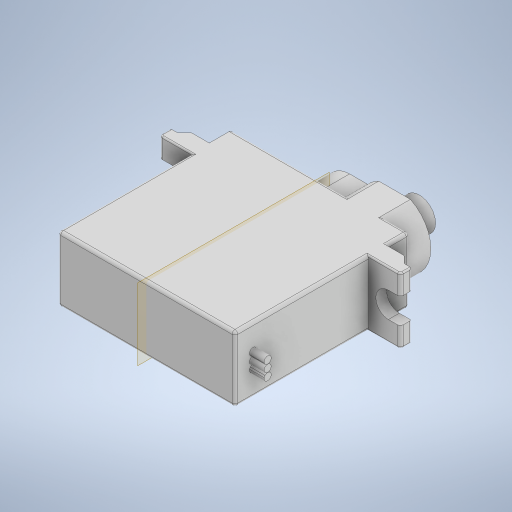
# Autodesk Inventor part: servo_stefan
Saved by Autodesk Inventor 2023 (Build 270158000, 158)
## iProperties
Created: 2023-04-06
Part Number: servo_stefan
Material: Ogólny
Document SubType Name: Modeling
Designer: Kamil
Density: 1 g/cm^3
Appearance: Domyślna
Author: Kamil
Autodesk Inventor part; units mm, degrees
ref_plane "YZ Plane" through (0, 0, 0) normal (1, 0, 0) x (0, 1, 0)
ref_plane "XZ Plane" through (0, 0, 0) normal (0, 1, 0) x (-1, 0, 0)
ref_plane "XY Plane" through (0, 0, 0) normal (0, 0, 1) x (1, 0, 0)
sketch "Szkic1" plane through (0, 0, 0) normal (0, 1, 0) x (-1, 0, 0)
  line L0 (0, 0) -> (24.4, 0)
  line L1 (24.4, 0) -> (24.4, -24)
  line L2 (24.4, -24) -> (0, -24)
  line L3 (0, -24) -> (0, 0)
  dimension "d0" = 24.4
  dimension "d1" = 24
  constraints: 8 end point, 2 parallel, 1 horizontal, 1 perpendicular
  measures "d0" distance of L1.end L2.end
  measures "d1" distance of L0.end L1.end
extrude "Wyciągnięcie proste1" add sketch "Szkic1" along normal blind 9
sketch "Szkic2" plane through (-24.4, 0, -24) normal (-1, 0, 0) x (0, 0, 1)
  line L0 (0, 0) -> (24, 0) projected
  line L1 (24, 0) -> (24, 9) projected
  line L2 (0, 9) -> (24, 9) projected
  line L3 (0, 0) -> (0, 9) projected
  line L4 (24, 0) -> (5.6, 0)
  line L5 (5.6, 0) -> (5.6, 9)
  line L6 (5.6, 9) -> (24, 9)
  line L7 (24, 9) -> (24, 0)
  line L8 (5.6, 9) -> (4.1, 9)
  line L9 (4.1, 9) -> (4.1, 0)
  line L10 (4.1, 0) -> (5.6, 0)
  line L11 (5.6, 0) -> (5.6, 9)
  line L12 (5.6, 9) -> (3.14, 9)
  line L13 (3.14, 9) -> (3.14, 0)
  line L14 (3.14, 0) -> (5.6, 0)
  line L15 (5.6, 0) -> (5.6, 9)
  line L16 (3.14, 9) -> (4.1, 9)
  line L17 (4.1, 9) -> (4.1, 7.5)
  line L18 (4.1, 7.5) -> (3.14, 7.5)
  line L19 (3.14, 7.5) -> (3.14, 9)
  line L20 (3.14, 0) -> (4.1, 0)
  line L21 (4.1, 0) -> (4.1, 1.5)
  line L22 (4.1, 1.5) -> (3.14, 1.5)
  line L23 (3.14, 1.5) -> (3.14, 0)
  dimension "d4" = 18.4
  dimension "d5" = 1.5
  dimension "d6" = 2.46
  dimension "d7" = 1.5
  dimension "d8" = 1.5
  constraints: 40 end point, 10 parallel, 5 horizontal, 5 perpendicular, 5 point on line
  measures "d4" distance of L5.end L6.end
  measures "d5" distance of L10.end L9.end
  measures "d6" distance of L14.end L13.end
  measures "d7" distance of L16.end L17.end
  measures "d8" distance of L21.end L20.end
extrude "Wyciągnięcie proste2" add sketch "Szkic2" along normal blind 4.4 contours L13 L22 L9 L0 | L9 L2 L5 L0 | L2 L9 L18 L13
sketch "Szkic3" plane through (-24.4, 1.5, -19.9) normal (0, 0, -1) x (-1, 0, 0)
  line L0 (0, 0) -> (0, 6) projected
  line L1 (0, 0) -> (4.4, 0) projected
  line L2 (4.4, 6) -> (4.4, 0) projected
  line L3 (0, 6) -> (4.4, 6) projected
  line L4 (0, -1.5) -> (0, 7.5) projected
  line L5 (0, 3) -> (1, 3)
  line L6 (1, 3) -> (4.5, 3)
  circle A0 centre (2.75, 3) radius 1.75
  line L7 (2.75, 4.75) -> (7.5825, 4.75)
  line L8 (2.75, 1.25) -> (9.2722, 1.25)
  point P0 (-24.4, -1.5)
  point P1 (4.4, 4.75)
  point P2 (4.4, 1.25)
  dimension "d11" = 1
  dimension "d12" = 3.5
  constraints: 8 end point, 3 horizontal, 3 point on circle, 2 midpoint, 2 tangent, 1 centre point, 1 point on line
  measures "d11" distance of L5.start L5.end
  measures "d12" distance of L5.end L6.end
extrude "Wyciągnięcie proste3" cut sketch "Szkic3" against normal through all contours A0 L2 L6 | L6 L2 A0 | L8 A0 L2 | L7 L2 A0 picked at (2.148, 3.1298) picked at (2.148, 2.8702)
sketch "Szkic4" plane through (0, 0, 0) normal (0, -1, 0) x (1, 0, 0)
  line L0 (0, -24) -> (-24.4, -24) projected
  line L1 (0, 0) -> (0, -24) projected
  line L2 (-24.4, 0) -> (0, 0) projected
  line L3 (-24.4, -18.4) -> (-24.4, 0) projected
  line L4 (-24.4, -18.4) -> (-28.8, -18.4) projected
  line L5 (-28.8, -20.86) -> (-28.8, -18.4) projected
  line L6 (-24.4, -20.86) -> (-28.8, -20.86) projected
  line L7 (-24.4, -24) -> (-24.4, -20.86) projected
  line L8 (-24.4, -19.9) -> (-28.8, -19.9) projected
  line L9 (-28.8, -19.9) -> (-27.8, -19.9)
  line L10 (-27.8, -19.9) -> (-26.84, -20.86)
  line L11 (-24.4, -20.86) -> (-28.8, -20.86) projected
  dimension "d15" = 1
  dimension "d16" = 135
  constraints: 4 end point, 2 point on line
  measures "d15" distance of L8.end L9.end
  measures "d16" angle of L9 L10
extrude "Wyciągnięcie proste4" cut sketch "Szkic4" against normal through all contours L6 L5 L8 L10
ref_plane "Płaszczyzna konstrukcyjna1" through (-12.2, 0, 0) normal (1, 0, 0) x (0, 0, -1)
mirror "Odbij1" about plane through (-12.2, 0, 0) normal (1, 0, 0)
sketch "Szkic5" plane through (0, 0, -24) normal (0, 0, -1) x (-1, 0, 0)
  line L0 (0, 0) -> (24.4, 0) projected
  line L1 (24.4, 0) -> (24.4, 9) projected
  line L2 (0, 9) -> (24.4, 9) projected
  line L3 (0, 0) -> (0, 9) projected
  line L4 (0, 0) -> (0, 9) projected
  line L5 (0, 4.5) -> (1, 4.5)
  line L6 (1, 4.5) -> (11, 4.5)
  circle A0 centre (6, 4.5) radius 5
  line L7 (11, 4.5) -> (12.2, 4.5)
  circle A1 centre (12.2, 4.5) radius 3.35
  line L8 (12.2, 7.85) -> (7.6364, 7.85)
  line L9 (12.2, 1.15) -> (7.9806, 1.15)
  point P0 (9.7118, 7.85)
  point P1 (8.1794, 9)
  point P2 (3.8206, 9)
  point P3 (3.8206, 0)
  point P4 (8.1794, 0)
  point P5 (9.7118, 1.15)
  dimension "d19" = 1
  dimension "d20" = 10
  dimension "d22" = 6.7
  constraints: 10 end point, 4 horizontal, 2 coincident, 2 midpoint, 2 point on circle, 2 tangent, 1 centre point, 1 parallel, 3 other
  measures "d19" distance of L5.start L5.end
  measures "d20" distance of L5.end L6.end
  measures "d22" diameter of A1
extrude "Wyciągnięcie proste5" add sketch "Szkic5" along normal blind 4 contours A0 L6 A1 L0 | A0 L2 A1 L6 | A0 A1 L9 | A1 A0 L6 | L6 A0 A1 | A0 A1 | A0 L8 A1
sketch "Szkic6" plane through (0, 0, -28) normal (0, 0, -1) x (-1, 0, 0)
  arc A0 (9.7118, 7.85) -> (8.1794, 9) centre (6, 4.5) ccw projected
  line L0 (8.1794, 9) -> (3.8206, 9) projected
  arc A1 (3.8206, 9) -> (3.8206, 0) centre (6, 4.5) ccw projected
  line L1 (3.8206, 0) -> (8.1794, 0) projected
  arc A2 (8.1794, 0) -> (9.7118, 1.15) centre (6, 4.5) ccw projected
  line L2 (9.7118, 1.15) -> (12.2, 1.15) projected
  arc A3 (12.2, 1.15) -> (12.2, 7.85) centre (12.2, 4.5) ccw projected
  line L3 (12.2, 7.85) -> (9.7118, 7.85) projected
  circle A4 centre (6, 4.5) radius 2.25
  point P0 (0, 0)
  dimension "d25" = 4.5
  constraints: 1 centre point, 1 coincident
  measures "d25" diameter of A4
extrude "Wyciągnięcie proste6" add sketch "Szkic6" along normal blind 3.4 contours A4
fillet "Zaokrąglenie1" radius 0.4 20 edges at (0, 0, -9.2) (-24.4, 0, -9.2) (-24.4, 0, -22.43) (-16.2897, 0, -24) (-24.4, 4.5, -24) (-16.2897, 9, -24) (-1.9103, 0, -24) (0, 4.5, -24) (-1.9103, 9, -24) (0, 9, -9.2) (-24.4, 9, -9.2) (-24.4, 4.5, 0) (-12.2, 9, 0) (-12.2, 0, 0) (0, 4.5, 0) (0, 0, -22.43) (0, 9, -22.43) (3.4, 0.75, -19.9) (3.4, 8.25, -19.9) (-28.8, 1.375, -18.4)
fillet "Zaokrąglenie2" radius 0.4 3 edges at (4.4, 7.625, -18.4) (4.4, 1.375, -18.4) (-28.8, 7.625, -18.4)
fillet "Zaokrąglenie3" radius 0.2 18 edges at (-28.8, 7.625, -19.9) (-28.8, 1.375, -19.9) (4.4, 7.625, -19.9) (4.4, 1.375, -19.9) (-0.2, 0, -18.4) (4.4, 0, -19.35) (-0.2, 9, -18.4) (4.4, 9, -19.35) (-24.2, 0, -18.4) (-28.8, 0, -19.35) (-28.8, 9, -19.35) (-24.2, 9, -18.4) (-27.8, 0.75, -19.9) (-27.8, 8.25, -19.9) (2.44, 0.75, -20.86) (2.44, 8.25, -20.86) (-26.84, 8.25, -20.86) (-26.84, 0.75, -20.86)
sketch "Szkic7" plane through (0, 0.4, -18.4) normal (1, 0, 0) x (0, 0, -1)
  line L0 (0.2, 8.6) -> (-18, 8.6) projected
  line L1 (-18.4, -0.4) -> (-13.4, -0.4)
  line L2 (-13.4, -0.4) -> (-13.4, 8.6)
  line L3 (-13.4, 8.6) -> (-18.4, 8.6)
  line L4 (-18.4, 8.6) -> (-18.4, -0.4)
  circle A0 centre (-15.9, 5.1) radius 0.5
  line L5 (-15.9, 5.1) -> (-15.9, 4.1)
  line L6 (-15.9, 4.1) -> (-15.9, 3.1)
  circle A1 centre (-15.9, 4.1) radius 0.5
  circle A2 centre (-15.9, 3.1) radius 0.5
  line L7 (-13.4, 8.6) -> (-18.4, -0.4)
  line L8 (-18.4, 8.6) -> (-13.4, -0.4)
  point P0 (-15.9, 4.1)
  point P1 (-16.3823, 4.9681)
  point P2 (-16.2668, 4.7602)
  point P3 (-15.9, 4.6)
  point P4 (-15.5332, 4.7602)
  point P5 (-15.4177, 4.9681)
  point P6 (-15.4177, 3.2319)
  point P7 (-15.5332, 3.4398)
  point P8 (-15.9, 3.6)
  point P9 (-16.2668, 3.4398)
  point P10 (-16.3823, 3.2319)
  dimension "d31" = 5
  dimension "d32" = 1
  dimension "d33" = 1
  dimension "d34" = 1
  constraints: 16 end point, 3 centre point, 2 coincident, 2 parallel, 2 point on line, 1 horizontal, 1 midpoint, 1 perpendicular, 1 vertical
  measures "d31" distance of L3.end L2.end
  measures "d32" diameter of A0
  measures "d33" distance of L5.start L5.end
  measures "d34" distance of L5.end L6.end
extrude "Wyciągnięcie proste7" add sketch "Szkic7" along normal blind 2 contours L7 A0 L8 | A2 L7 L8 | A1 L7 L5 | L5 L8 A1 | A1 L8 L7 | A1 L7 L6 | L6 L8 A1 | L7 A1 L8
